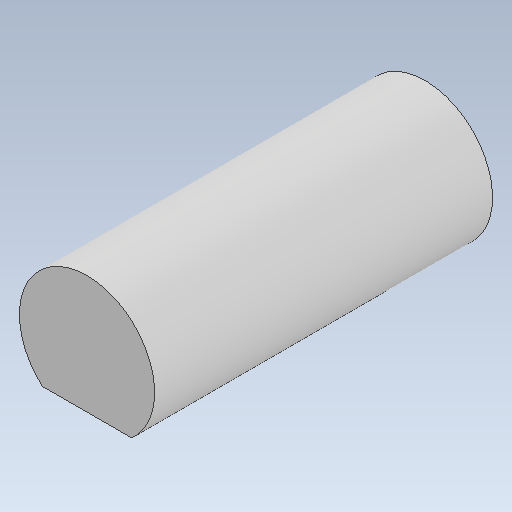
# Autodesk Inventor part: shaft
Saved by Autodesk Inventor 2021 (Build 250183000, 183)
## iProperties
Created: 2021-07-09
Part Number: shaft
Material: Generic
Document SubType Name: Modeling
Designer: TARUN
Density: 1 g/cm^3
Appearance: Default
Author: TARUN
Autodesk Inventor part; units mm, degrees
ref_plane "YZ Plane" through (0, 0, 0) normal (1, 0, 0) x (0, 1, 0)
ref_plane "XZ Plane" through (0, 0, 0) normal (0, 1, 0) x (-1, 0, 0)
ref_plane "XY Plane" through (0, 0, 0) normal (0, 0, 1) x (1, 0, 0)
sketch "Sketch1" plane through (0, 0, 0) normal (0, 0, 1) x (1, 0, 0)
  arc A0 (2.6447, -3.0009) -> (-2.6447, -3.0009) centre (0, 0) ccw
  line L0 (0, 0) -> (-2.6447, -3.0009) construction
  line L1 (0, 0) -> (4, 0) construction
  line L2 (0, 0) -> (2.6447, -3.0009) construction
  line L3 (-2.6447, -3.0009) -> (2.6447, -3.0009)
  dimension "d3" = 4
  dimension "d4" = 131.39
  dimension "d5" = 82.78
  constraints: 8 end point, 2 point on circle, 1 centre point, 1 coincident, 1 equal length, 1 horizontal
  measures "d3" radius of A0
  measures "d4" angle of L0 L1
  measures "d5" angle of L0 L2
extrude "Extrusion1" add sketch "Sketch1" along normal blind 20
sketch "Sketch2" plane through (0, 0, 0) normal (0, 0, -1) x (-1, 0, 0)
  line L0 (2.6447, -3.0009) -> (-2.6447, -3.0009) projected
  arc A0 (2.6447, -3.0009) -> (-2.6447, -3.0009) centre (0, 0) ccw projected
  arc A1 (-2.6447, -3.0009) -> (2.6447, -3.0009) centre (0, 0) ccw
  line L1 (-2.6447, -3.0009) -> (2.6447, -3.0009)
  constraints: 2 end point, 2 point on circle, 1 centre point, 1 collinear
extrude "Extrusion2" add sketch "Sketch2" against normal blind 5 contours A1 L0
body "Solid1"
